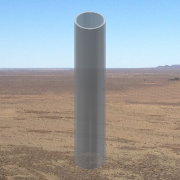
# Autodesk Inventor part: 2f1mast
Saved by Autodesk Inventor 2014 SP1 (Build 180222100, 222)
## iProperties
Company: HERA Project
Created: 2013-05-22
Part Number: 2f1mast
Material: Glass
Document SubType Name: Modeling
Designer: Rich Bradley
Density: 2.18 g/cm^3
Description: Feed mast
Mass: 1508.6 g
Surface Area: 2551.42 cm^2
Volume: 692.018 cm^3
Appearance: Clear
Author: David DeBoer
Title: Feed mast
Autodesk Inventor part; units mm, degrees
ref_plane "YZ Plane" through (0, 0, 0) normal (1, 0, 0) x (0, 1, 0)
ref_plane "XZ Plane" through (0, 0, 0) normal (0, 1, 0) x (-1, 0, 0)
ref_plane "XY Plane" through (0, 0, 0) normal (0, 0, 1) x (1, 0, 0)
sketch "Sketch1" plane through (0, 0, 0) normal (0, 1, 0) x (-1, 0, 0)
  circle A0 centre (0, 0) radius 44.45
  circle A1 centre (0, 0) radius 38.9636
  dimension "d0" = 88.9
  dimension "d1" = 5.4864
  constraints: 2 centre point, 1 coincident
  measures "d0" diameter of A0
  measures "d1" radial gap between concentric circles of A1 A0
extrude "Extrusion1" add sketch "Sketch1" along normal blind 481.33
body "Solid1"
